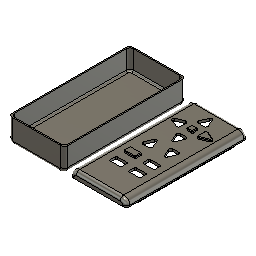
northreach_1_v2 (Autodesk Fusion 360 design; units mm, degrees)
Autodesk Fusion 360 part; units mm, degrees
note: some values were not read from the file. Set by a fixed rule: which sketch regions a step uses.
sketch "MainBodyBase" plane through (0, 0, 0) normal (0, 1, 0) x (1, 0, 0)
  line L0 (-22.5, 50) -> (22.5, 50)
  line L1 (22.5, 50) -> (22.5, -50)
  line L2 (22.5, -50) -> (-22.5, -50)
  line L3 (-22.5, -50) -> (-22.5, 50)
  line L4 (-22.5, 50) -> (22.5, -50) construction
  line L5 (22.5, 50) -> (-22.5, -50) construction
  line L6 (-23.5, 51) -> (23.5, 51)
  line L7 (23.5, 51) -> (23.5, -51)
  line L8 (23.5, -51) -> (-23.5, -51)
  line L9 (-23.5, -51) -> (-23.5, 51)
  line L10 (-23.5, 51) -> (23.5, -51) construction
  line L11 (23.5, 51) -> (-23.5, -51) construction
  dimension "d1" = 45
  dimension "d2" = 100
  dimension "d3" = 47
  dimension "d4" = 102
  constraint horizontal L0
  constraint perpendicular L0 L1
  constraint parallel L0 L2
  constraint parallel L1 L3
  constraint coincident L4 origin
  constraint coincident L5 origin
  constraint horizontal L6
  constraint perpendicular L6 L7
  constraint parallel L6 L8
  constraint parallel L7 L9
  constraint coincident L10 origin
  constraint coincident L11 origin
  measures "d1" distance of L1.end L2.end
  measures "d2" distance of L0.end L1.end
  measures "d3" distance of L7.end L8.end
  measures "d4" distance of L6.end L7.end
extrude "Extrude1" add sketch "MainBodyBase" along normal blind 3 contours L0 L1 L2 L3 makes body 1
extrude "Extrude2" add sketch "MainBodyBase" along normal blind 20 bodies 1
fillet "Fillet1" radius 4 2 edges at (-23.5, 0, 0) (23.5, 0, 0) on bodies 1
sketch "TopCoverBase" plane through (0, 0, 0) normal (0, 1, 0) x (1, 0, 0)
  line L0 (46.5, 51) -> (93.5, 51)
  line L1 (93.5, 51) -> (93.5, -51)
  line L2 (93.5, -51) -> (46.5, -51)
  line L3 (46.5, -51) -> (46.5, 51)
  line L4 (46.5, 51) -> (93.5, -51) construction
  line L5 (93.5, 51) -> (46.5, -51) construction
  line L6 (48.5, 50) -> (91.5, 50)
  line L7 (91.5, 50) -> (91.5, -50)
  line L8 (91.5, -50) -> (48.5, -50)
  line L9 (48.5, -50) -> (48.5, 50)
  line L10 (48.5, 50) -> (91.5, -50) construction
  line L11 (91.5, 50) -> (48.5, -50) construction
  line L12 (47.5, 50) -> (47.5, -50)
  line L13 (48.5, -50) -> (48.5, 50)
  line L14 (92.5, -50) -> (92.5, 50)
  line L15 (91.5, 50) -> (91.5, -50)
  line L16 (47.5, 39.9985) -> (48.5, 39.9985)
  line L17 (47.5, -40) -> (48.5, -40)
  line L18 (91.5, -40) -> (92.5, -40)
  line L19 (91.5, 39.9985) -> (92.5, 39.9985)
  point P0 (70, 0)
  point P1 (70, 0)
  dimension "d22" = 47
  dimension "d23" = 102
  dimension "d24" = 43
  dimension "d25" = 100
  constraint horizontal L0
  constraint perpendicular L0 L1
  constraint parallel L0 L2
  constraint parallel L1 L3
  constraint coincident L4 P1
  constraint coincident L5 P1
  constraint horizontal L6
  constraint perpendicular L6 L7
  constraint parallel L6 L8
  constraint parallel L7 L9
  constraint coincident L10 P1
  constraint coincident L11 P1
  constraint coincident P1 P0
  constraint vertical L12
  constraint vertical L13
  constraint vertical L14
  constraint vertical L15
  constraint coincident L12 L16.start
  constraint coincident L13 L16.end
  constraint perpendicular L13 L16
  constraint coincident L12 L17.start
  constraint coincident L13 L17.end
  constraint perpendicular L13 L17
  constraint coincident L15 L18.start
  constraint coincident L14 L18.end
  constraint perpendicular L14 L18
  constraint coincident L7 L19.start
  constraint coincident L14 L19.end
  constraint perpendicular L14 L19
  measures "d22" distance of L1.end L2.end
  measures "d23" distance of L0.end L1.end
  measures "d24" distance of L7.end L8.end
  measures "d25" distance of L6.end L7.end
extrude "Extrude7" add sketch "TopCoverBase" along normal blind 2 separate body contours L6 L7 L8 L9 L13 L15 makes body 2
extrude "Extrude8" add sketch "TopCoverBase" along normal blind 6 contours L0 L1 L2 L3 | L9 L12 L13 L16 L17 | L7 L14 L15 L18 L19 bodies 2
extrude "Extrude9" add sketch "TopCoverBase" along normal blind 7.5 contours L9 L12 L13 L16 L17 | L7 L14 L15 L18 L19 bodies 2
fillet "Fillet2" radius 5 2 edges at (46.5, 0, 0) (93.5, 0, 0) on bodies 2
fillet "Fillet2" radius 3 2 edges at (91.5, 2, 0) (48.5, 2, 0) on bodies 2
move_body "Move1" bodies 2 to x (-1, 0, 0) y (0, -1, 0) z (0, 0, 1) at (122, 7.5, 0)
sketch "ButtonHoles" plane through (0, 7.5, 0) normal (0, 1, 0) x (-1, 0, 0)
  line L0 (-33.5, -51) -> (-33.5, 51)
  line L1 (-33.5, 51) -> (-70.5, 51)
  line L2 (-70.5, 51) -> (-70.5, -51)
  line L3 (-70.5, -51) -> (-33.5, -51)
  arc A0 (-39, 16.25) -> (-39.75, 17) centre (-39.75, 16.25) ccw
  line L4 (-49, 14) -> (-55, 14)
  arc A1 (-50.25, -30.5) -> (-49.5, -29.75) centre (-50.25, -29.75) ccw
  line L5 (-39.75, 11) -> (-48.25, 11)
  arc A2 (-55, 16.25) -> (-55.75, 17) centre (-55.75, 16.25) ccw
  line L6 (-46, 14) -> (-42, 14)
  line L7 (-53.75, -30.5) -> (-50.25, -30.5)
  line L8 (-54.5, -26.25) -> (-54.5, -29.75)
  line L9 (-49.5, -25.5) -> (-54.5, -30.5) construction
  arc A3 (-65, 11.75) -> (-64.25, 11) centre (-64.25, 11.75) ccw
  line L10 (-65, 11) -> (-55, 17) construction
  line L11 (-39, 16.25) -> (-39, 11.75)
  line L12 (-48.25, 17) -> (-39.75, 17)
  line L13 (-65, 23) -> (-55, 29) construction
  line L14 (-62, 26) -> (-58, 26)
  line L15 (-41.4931, 3.0384) -> (-46.5069, 3.0384)
  line L16 (-39, 28.25) -> (-39, 23.75)
  line L17 (-55.75, 23) -> (-64.25, 23)
  arc A4 (-39.75, 11) -> (-39, 11.75) centre (-39.75, 11.75) ccw
  line L18 (-49, 23) -> (-39, 29) construction
  line L19 (-39.75, 23) -> (-48.25, 23)
  arc A5 (-64.25, 29) -> (-65, 28.25) centre (-64.25, 28.25) ccw
  line L20 (-55, 11) -> (-65, 17) construction
  arc A6 (-49.5, -26.25) -> (-50.25, -25.5) centre (-50.25, -26.25) ccw
  line L21 (-49, 11) -> (-39, 17) construction
  arc A7 (-49, 23.75) -> (-48.25, 23) centre (-48.25, 23.75) ccw
  line L22 (-47.8763, 0.9617) -> (-45.1295, -5.4475)
  line L23 (-55, 28.25) -> (-55, 23.75)
  line L24 (-49, 26) -> (-55, 26)
  arc A8 (-47.8763, 0.9617) -> (-46.5069, 3.0384) centre (-46.5069, 1.5486) cw
  line L25 (-42.8705, -5.4475) -> (-40.1237, 0.9617)
  line L26 (-55, 23) -> (-65, 29) construction
  arc A9 (-55, 28.25) -> (-55.75, 29) centre (-55.75, 28.25) ccw
  line L27 (-54.5, -25.5) -> (-49.5, -30.5) construction
  line L28 (-65, 23.75) -> (-65, 28.25)
  line L29 (-46, 26) -> (-42, 26)
  line L30 (-64.25, 17) -> (-55.75, 17)
  line L31 (-39, 11) -> (-49, 17) construction
  arc A10 (-54.5, -29.75) -> (-53.75, -30.5) centre (-53.75, -29.75) ccw
  line L32 (-50.25, -25.5) -> (-53.75, -25.5)
  arc A11 (-53.75, -25.5) -> (-54.5, -26.25) centre (-53.75, -26.25) ccw
  line L33 (-44, 12) -> (-44, 16)
  arc A12 (-49, 11.75) -> (-48.25, 11) centre (-48.25, 11.75) ccw
  line L34 (-60, 24) -> (-60, 28)
  line L35 (-65, 11.75) -> (-65, 16.25)
  line L36 (-44, 24) -> (-44, 28)
  line L37 (-39, 23) -> (-49, 29) construction
  line L38 (-62, 14) -> (-58, 14)
  line L39 (-49.5, -29.75) -> (-49.5, -26.25)
  line L40 (-60, 12) -> (-60, 16)
  arc A13 (-64.25, 17) -> (-65, 16.25) centre (-64.25, 16.25) ccw
  line L41 (-49, 11.75) -> (-49, 16.25)
  arc A14 (-65, 23.75) -> (-64.25, 23) centre (-64.25, 23.75) ccw
  arc A15 (-41.4931, 3.0384) -> (-40.1237, 0.9617) centre (-41.4931, 1.5486) cw
  arc A16 (-48.25, 17) -> (-49, 16.25) centre (-48.25, 16.25) ccw
  arc A17 (-39, 28.25) -> (-39.75, 29) centre (-39.75, 28.25) ccw
  line L42 (-44, -6.1923) -> (-44, 3.0384)
  line L43 (-49, 23.75) -> (-49, 28.25)
  arc A18 (-55.75, 11) -> (-55, 11.75) centre (-55.75, 11.75) ccw
  arc A19 (-39.75, 23) -> (-39, 23.75) centre (-39.75, 23.75) ccw
  line L44 (-48.25, 29) -> (-39.75, 29)
  line L45 (-55.75, 11) -> (-64.25, 11)
  arc A20 (-48.25, 29) -> (-49, 28.25) centre (-48.25, 28.25) ccw
  arc A21 (-42.8705, -5.4475) -> (-45.1295, -5.4475) centre (-44, -4.9635) cw
  line L46 (-64.25, 29) -> (-55.75, 29)
  arc A22 (-55.75, 23) -> (-55, 23.75) centre (-55.75, 23.75) ccw
  line L47 (-55, 16.25) -> (-55, 11.75)
  line L48 (-42, 16) -> (-46, 16) construction
  line L49 (-46, 16) -> (-46, 12) construction
  line L50 (-46, 12) -> (-42, 12) construction
  line L51 (-42, 12) -> (-42, 16) construction
  line L52 (-42, 28) -> (-46, 28) construction
  line L53 (-46, 28) -> (-46, 24) construction
  line L54 (-46, 24) -> (-42, 24) construction
  line L55 (-42, 24) -> (-42, 28) construction
  line L56 (-58, 16) -> (-62, 16) construction
  line L57 (-62, 16) -> (-62, 12) construction
  line L58 (-62, 12) -> (-58, 12) construction
  line L59 (-58, 12) -> (-58, 16) construction
  line L60 (-58, 28) -> (-62, 28) construction
  line L61 (-62, 28) -> (-62, 24) construction
  line L62 (-62, 24) -> (-58, 24) construction
  line L63 (-58, 24) -> (-58, 28) construction
  line L64 (-44, -1.577) -> (-60, -1.577)
  line L65 (-41.4931, 3.0384) -> (-46.5069, 3.0384)
  line L66 (-44, -6.1923) -> (-44, 3.0384)
  arc A23 (-47.8763, 0.9617) -> (-46.5069, 3.0384) centre (-46.5069, 1.5486) cw
  arc A24 (-42.8705, -5.4475) -> (-45.1295, -5.4475) centre (-44, -4.9635) cw
  line L67 (-42.8705, -5.4475) -> (-40.1237, 0.9617)
  arc A25 (-41.4931, 3.0384) -> (-40.1237, 0.9617) centre (-41.4931, 1.5486) cw
  line L68 (-47.8763, 0.9617) -> (-45.1295, -5.4475)
  line L69 (-62.5069, -6.1923) -> (-57.4931, -6.1923)
  line L70 (-60, 3.0384) -> (-60, -6.1923)
  arc A26 (-56.1237, -4.1156) -> (-57.4931, -6.1923) centre (-57.4931, -4.7025) cw
  arc A27 (-61.1295, 2.2936) -> (-58.8705, 2.2936) centre (-60, 1.8095) cw
  line L71 (-61.1295, 2.2936) -> (-63.8763, -4.1156)
  arc A28 (-62.5069, -6.1923) -> (-63.8763, -4.1156) centre (-62.5069, -4.7025) cw
  line L72 (-56.1237, -4.1156) -> (-58.8705, 2.2936)
  line L73 (-52, -11.2693) -> (-52, -20.5)
  line L74 (-53.1295, -12.0141) -> (-55.8763, -18.4233)
  arc A29 (-48.1237, -18.4233) -> (-49.4931, -20.5) centre (-49.4931, -19.0102) cw
  line L75 (-48.1237, -18.4233) -> (-50.8705, -12.0141)
  arc A30 (-54.5069, -20.5) -> (-55.8763, -18.4233) centre (-54.5069, -19.0102) cw
  line L76 (-54.5069, -20.5) -> (-49.4931, -20.5)
  arc A31 (-53.1295, -12.0141) -> (-50.8705, -12.0141) centre (-52, -12.4982) cw
  line L77 (-68.7307, -28) -> (-59.5, -28)
  line L78 (-67.9859, -29.1295) -> (-61.5767, -31.8763)
  arc A32 (-61.5767, -24.1237) -> (-59.5, -25.4931) centre (-60.9898, -25.4931) cw
  line L79 (-61.5767, -24.1237) -> (-67.9859, -26.8705)
  arc A33 (-59.5, -30.5069) -> (-61.5767, -31.8763) centre (-60.9898, -30.5069) cw
  line L80 (-59.5, -30.5069) -> (-59.5, -25.4931)
  arc A34 (-67.9859, -29.1295) -> (-67.9859, -26.8705) centre (-67.5019, -28) cw
  line L81 (-35.2693, -28) -> (-44.5, -28)
  line L82 (-36.0141, -26.8705) -> (-42.4233, -24.1237)
  arc A35 (-42.4233, -31.8763) -> (-44.5, -30.5069) centre (-43.0102, -30.5069) cw
  line L83 (-42.4233, -31.8763) -> (-36.0141, -29.1295)
  arc A36 (-44.5, -25.4931) -> (-42.4233, -24.1237) centre (-43.0102, -25.4931) cw
  line L84 (-44.5, -25.4931) -> (-44.5, -30.5069)
  arc A37 (-36.0141, -26.8705) -> (-36.0141, -29.1295) centre (-36.4981, -28) cw
  line L85 (-52, -44.7307) -> (-52, -35.5)
  line L86 (-50.8705, -43.9859) -> (-48.1237, -37.5767)
  arc A38 (-55.8763, -37.5767) -> (-54.5069, -35.5) centre (-54.5069, -36.9898) cw
  line L87 (-55.8763, -37.5767) -> (-53.1295, -43.9859)
  arc A39 (-49.4931, -35.5) -> (-48.1237, -37.5767) centre (-49.4931, -36.9898) cw
  line L88 (-49.4931, -35.5) -> (-54.5069, -35.5)
  arc A40 (-50.8705, -43.9859) -> (-53.1295, -43.9859) centre (-52, -43.5019) cw
  point P0 (-44, 26)
  point P1 (-60, 14)
  point P2 (-44, 3.0384)
  point P3 (-52.0007, 8.4459)
  point P4 (-44, 14)
  point P5 (-41.5, 10)
  point P6 (-44, 14)
  point P7 (-41.5, 22)
  point P8 (-44, 26)
  point P9 (-52, 14)
  point P10 (-44, -1.577)
  point P11 (-52, 26)
  point P12 (-60, 14)
  point P13 (-52, -28)
  point P14 (-60, 26)
  point P15 (-60, 26)
  point P16 (-52, -1.577)
  point P17 (-44, 3.0384)
  point P18 (-44, -1.577)
  point P19 (-44, -1.577)
  point P20 (-60, -6.1923)
  point P21 (-60, -1.577)
  point P22 (-60, -1.577)
  point P23 (-52, -15.8847)
  point P24 (-52, -20.5)
  point P25 (-52, -15.8847)
  point P26 (-52, -15.8847)
  point P27 (-64.1153, -28)
  point P28 (-59.5, -28)
  point P29 (-64.1153, -28)
  point P30 (-64.1153, -28)
  point P31 (-39.8847, -28)
  point P32 (-44.5, -28)
  point P33 (-39.8847, -28)
  point P34 (-39.8847, -28)
  point P35 (-52, -40.1153)
  point P36 (-52, -35.5)
  point P37 (-52, -40.1153)
  point P38 (-52, -40.1153)
  dimension "d46" = 3
  dimension "d47" = 0
  dimension "d50" = 3
  dimension "d51" = 0
  dimension "d48" = 3
  dimension "d49" = 0
  dimension "d52" = 3
  dimension "d53" = 0
  dimension "d55" = 0.75
  dimension "d56" = 10
  dimension "d57" = 6
  dimension "d58" = 10
  dimension "d59" = 6
  dimension "d60" = 6
  dimension "d61" = 0.75
  dimension "d62" = 10
  dimension "d63" = 6
  dimension "d64" = 10
  dimension "d65" = 6
  dimension "d66" = 6
  dimension "d67" = 0.75
  text T0 "1" font "Arial" height 3 align centre middle in box 4 x 4 at (-42, 16) x (-1, 0) y (0, -1) spacing 1
  text T1 "3" font "Arial" height 3 align centre middle in box 4 x 4 at (-42, 28) x (-1, 0) y (0, -1) spacing 1
  text T2 "2" font "Arial" height 3 align centre middle in box 4 x 4 at (-58, 16) x (-1, 0) y (0, -1) spacing 1
  text T3 "4" font "Arial" height 3 align centre middle in box 4 x 4 at (-58, 28) x (-1, 0) y (0, -1) spacing 1
  constraint horizontal L32
  constraint perpendicular L8 L32
  constraint parallel L7 L32
  constraint parallel L8 L39
  constraint coincident P13 L9
  constraint coincident P13 L27
  constraint coincident L9.end L7
  constraint coincident L9.end L8
  constraint tangent L7 A10
  constraint tangent L8 A10
  constraint coincident L27.end L7
  constraint coincident L27.end L39
  constraint tangent A1 L7
  constraint tangent A1 L39
  constraint equal A1 A10
  constraint coincident L9.start L39
  constraint coincident L9.start L32
  constraint tangent A6 L39
  constraint tangent A6 L32
  constraint equal A6 A10
  constraint coincident L27.start L32
  constraint coincident L27.start L8
  constraint tangent L32 A11
  constraint tangent L8 A11
  constraint equal A10 A11
  constraint tangent L15 A8
  constraint tangent L22 A8
  constraint tangent L15 A15
  constraint tangent L25 A15
  constraint tangent L22 A21
  constraint tangent L25 A21
  constraint midpoint P17 L15
  constraint midpoint L42.start A21
  constraint coincident P17 P2
  constraint perpendicular L15 L42
  constraint midpoint P19 L42
  constraint horizontal L45
  constraint perpendicular L35 L45
  constraint parallel L30 L45
  constraint parallel L35 L47
  constraint horizontal L5
  constraint perpendicular L5 L41
  constraint parallel L5 L12
  constraint parallel L11 L41
  constraint midpoint P9 L4
  constraint tangent L11 A4
  constraint tangent L5 A4
  constraint tangent A0 L11
  constraint tangent A0 L12
  constraint equal A0 A4
  constraint coincident L4.start L41
  constraint tangent L12 A16
  constraint tangent L41 A16
  constraint equal A4 A16
  constraint tangent L5 A12
  constraint tangent A12 L41
  constraint equal A4 A12
  constraint coincident L4.end L47
  constraint coincident L20.start L47
  constraint tangent A18 L45
  constraint tangent A18 L47
  constraint equal A4 A18
  constraint coincident L10.end L47
  constraint tangent A2 L47
  constraint tangent A2 L30
  constraint equal A2 A4
  constraint coincident L20.end L30
  constraint tangent L30 A13
  constraint tangent L35 A13
  constraint equal A4 A13
  constraint tangent A3 L45
  constraint tangent A3 L35
  constraint equal A3 A4
  constraint horizontal L17
  constraint perpendicular L17 L28
  constraint parallel L17 L46
  constraint parallel L23 L28
  constraint horizontal L19
  constraint perpendicular L19 L43
  constraint parallel L19 L44
  constraint parallel L16 L43
  constraint midpoint P11 L24
  constraint tangent L16 A19
  constraint tangent L19 A19
  constraint tangent L16 A17
  constraint tangent A17 L44
  constraint equal A17 A19
  constraint coincident L24.start L43
  constraint tangent L44 A20
  constraint tangent L43 A20
  constraint equal A19 A20
  constraint tangent L19 A7
  constraint tangent A7 L43
  constraint equal A7 A19
  constraint coincident L24.end L23
  constraint coincident L26.start L23
  constraint tangent L17 A22
  constraint tangent L23 A22
  constraint equal A19 A22
  constraint coincident L13.end L23
  constraint tangent L23 A9
  constraint tangent A9 L46
  constraint equal A9 A19
  constraint coincident L26.end L46
  constraint tangent A5 L46
  constraint tangent A5 L28
  constraint equal A5 A19
  constraint tangent L17 A14
  constraint tangent L28 A14
  constraint equal A14 A19
  constraint midpoint L33.start L50
  constraint midpoint L33.end L48
  constraint midpoint L6.start L49
  constraint midpoint L6.end L51
  constraint midpoint P6 L6
  constraint midpoint L40.start L58
  constraint midpoint L40.end L56
  constraint midpoint L38.start L57
  constraint midpoint L38.end L59
  constraint midpoint P1 L38
  constraint midpoint L36.start L54
  constraint midpoint L36.end L52
  constraint midpoint L29.start L53
  constraint midpoint L29.end L55
  constraint midpoint P8 L29
  constraint midpoint L34.start L62
  constraint midpoint L34.end L60
  constraint midpoint L14.start L61
  constraint midpoint L14.end L63
  constraint midpoint P15 L14
  constraint coincident P19 P18
  constraint tangent L65 A23
  constraint tangent A23 L68
  constraint tangent L65 A25
  constraint tangent L67 A25
  constraint tangent A24 L68
  constraint tangent A24 L67
  constraint midpoint P17 L65
  constraint midpoint L42.start A24
  constraint perpendicular L65 L66
  constraint midpoint P19 L66
  constraint tangent L69 A26
  constraint tangent A26 L72
  constraint tangent L69 A28
  constraint tangent L71 A28
  constraint tangent A27 L72
  constraint tangent A27 L71
  constraint midpoint P20 L69
  constraint midpoint L70.start A27
  constraint coincident P20 L70.end
  constraint perpendicular L69 L70
  constraint midpoint P22 L70
  constraint coincident P22 P21
  constraint tangent A29 L76
  constraint tangent A29 L75
  constraint tangent A30 L76
  constraint tangent L74 A30
  constraint tangent L75 A31
  constraint tangent L74 A31
  constraint midpoint P24 L76
  constraint midpoint L73.start A31
  constraint coincident P24 L73.end
  constraint perpendicular L73 L76
  constraint midpoint P26 L73
  constraint coincident P26 P25
  constraint tangent A32 L80
  constraint tangent A32 L79
  constraint tangent A33 L80
  constraint tangent L78 A33
  constraint tangent L79 A34
  constraint tangent L78 A34
  constraint midpoint P28 L80
  constraint midpoint L77.start A34
  constraint coincident P28 L77.end
  constraint perpendicular L77 L80
  constraint midpoint P30 L77
  constraint coincident P30 P29
  constraint tangent A35 L84
  constraint tangent A35 L83
  constraint tangent A36 L84
  constraint tangent L82 A36
  constraint tangent L83 A37
  constraint tangent L82 A37
  constraint midpoint P32 L84
  constraint midpoint L81.start A37
  constraint coincident P32 L81.end
  constraint perpendicular L81 L84
  constraint midpoint P34 L81
  constraint coincident P34 P33
  constraint tangent A38 L88
  constraint tangent A38 L87
  constraint tangent A39 L88
  constraint tangent L86 A39
  constraint tangent L87 A40
  constraint tangent L86 A40
  constraint midpoint P36 L88
  constraint midpoint L85.start A40
  constraint coincident P36 L85.end
  constraint perpendicular L85 L88
  constraint midpoint P38 L85
  constraint coincident P38 P37
  measures "d55" radius of A10
  measures "d56" distance of L20.end L10.end
  measures "d57" distance of L20.end L10.start
  measures "d58" distance of L21.end L31.end
  measures "d59" distance of L21.start L31.end
  measures "d60" distance of L41 L47
  measures "d61" radius of A4
  measures "d62" distance of L13.end L26.end
  measures "d63" distance of L13.start L26.end
  measures "d64" distance of L37.end L18.end
  measures "d65" distance of L37.end L18.start
  measures "d66" distance of L23 L43
  measures "d67" radius of A19
extrude "Extrude10" cut sketch "ButtonHoles" sketch "ButtonHoles" against normal blind 32 contours A0 L5 L11 L12 A4 A12 L41 A16 | A1 L7 L8 A6 A10 L32 A11 L39 | A2 A3 L30 L35 A13 A18 L45 L47 | L15 L25 A15 L42 A21 L65 L66 A24 L67 A25 | L15 L22 A8 L42 L64 L65 L66 A23 L68 | L22 L42 A21 L64 L66 A24 L68 | L16 L19 A7 A17 L43 A19 L44 A20 | L17 A5 L23 A9 L28 A14 L46 A22 | L64 L69 L70 A26 L72 | L64 L70 A27 L72 | L69 L70 A27 L71 A28 | L73 A29 L75 L76 A31 | L73 L74 A30 L76 A31 | L77 A32 L79 L80 A34 | L77 L78 A33 L80 A34 | L81 A35 L83 L84 A37 | L81 L82 A36 L84 A37 | L85 A38 L87 L88 A40 | L85 L86 A39 L88 A40 of sketch 2 text T0 T1 T2 T3 bodies 2
fillet "Fillet4" radius 3 14 edges at (23.5, 12, 51) (22.3284, 1.1716, 51) (0, 0, 51) (-22.3284, 1.1716, 51) (-23.5, 12, 51) (-22.5, 11.5, 50) (22.5, 11.5, 50) (-23.5, 12, -51) (-22.3284, 1.1716, -51) (0, 0, -51) (22.3284, 1.1716, -51) (23.5, 12, -51) (22.5, 11.5, -50) (-22.5, 11.5, -50) on bodies 1
fillet "Fillet5" radius 3 10 edges at (28.5, 2, 51) (29.9645, 6.0355, 51) (52, 7.5, 51) (74.0355, 6.0355, 51) (75.5, 2, 51) (75.5, 2, -51) (74.0355, 6.0355, -51) (52, 7.5, -51) (29.9645, 6.0355, -51) (28.5, 2, -51) on bodies 2
fillet "Fillet6" radius 1.5 8 edges at (0, 3, -50) (-21.6213, 3, -49.1213) (-22.5, 3, 0) (-21.6213, 3, 49.1213) (0, 3, 50) (21.6213, 3, 49.1213) (22.5, 3, 0) (21.6213, 3, -49.1213) on bodies 1
sketch "TriangleButton" plane through (0, 0, 0) normal (0, 1, 0) x (1, 0, 0)
  line L0 (-60, 2.8999) -> (-60, -6.0539)
  line L1 (-61.0956, 2.1775) -> (-63.76, -4.0395)
  arc A0 (-56.24, -4.0395) -> (-57.5683, -6.0539) centre (-57.5683, -4.6087) cw
  line L2 (-56.24, -4.0395) -> (-58.9044, 2.1775)
  arc A1 (-62.4317, -6.0539) -> (-63.76, -4.0395) centre (-62.4317, -4.6087) cw
  line L3 (-62.4317, -6.0539) -> (-57.5683, -6.0539)
  arc A2 (-61.0956, 2.1775) -> (-58.9044, 2.1775) centre (-60, 1.7079) cw
  point P0 (-60, -1.577)
  point P1 (-60, -6.0539)
  point P2 (-60, -1.577)
  point P3 (-60, -1.577)
  constraint tangent A0 L3
  constraint tangent A0 L2
  constraint tangent A1 L3
  constraint tangent L1 A1
  constraint tangent L2 A2
  constraint tangent L1 A2
  constraint midpoint P1 L3
  constraint midpoint L0.start A2
  constraint coincident P1 L0.end
  constraint perpendicular L0 L3
  constraint midpoint P3 L0
  constraint coincident P3 P2
extrude "Extrude12" add sketch "TriangleButton" along normal blind 6 separate body makes body 3
move_body "Move7" bodies 3 to x (0, 0, 1) y (0, 1, 0) z (-1, 0, 0) at (-67.0351, 0, 60.9584)
move_body "Move8" bodies 3 to x (1, 0, 0) y (0, 1, 0) z (0, 0, 1) at (132.7274, 1.5, -28.9584)
move_body "Move9" bodies 3 to x (1, 0, 0) y (0, 1, 0) z (0, 0, 1) at (-127, 0, 0)
ref_plane "WorkPlane1" through (-62.8847, 3.5, -28) normal (0, 1, 0) x (0, 0, 1)
sketch "TriangleButtonLip" plane through (0, 3.5, 0) normal (0, 1, 0) x (1, 0, 0)
  line L0 (-65.3472, 24.24) -> (-59.1302, 26.9044)
  arc A0 (-59.1302, 26.9044) -> (-59.1302, 29.0956) centre (-59.5997, 28) ccw
  line L1 (-59.1302, 29.0956) -> (-65.3472, 31.76)
  arc A1 (-65.3472, 31.76) -> (-67.3615, 30.4317) centre (-65.9164, 30.4317) ccw
  line L2 (-67.3615, 30.4317) -> (-67.3615, 25.5683)
  arc A2 (-67.3615, 25.5683) -> (-65.3472, 24.24) centre (-65.9164, 25.5683) ccw
  line L3 (-58.7363, 30.0147) -> (-64.9533, 32.6791)
  arc A3 (-64.9533, 32.6791) -> (-68.3615, 30.4317) centre (-65.9164, 30.4317) ccw
  line L4 (-68.3615, 30.4317) -> (-68.3615, 25.5683)
  arc A4 (-68.3615, 25.5683) -> (-64.9533, 23.3209) centre (-65.9164, 25.5683) ccw
  line L5 (-64.9533, 23.3209) -> (-58.7363, 25.9853)
  arc A5 (-58.7363, 25.9853) -> (-58.7363, 30.0147) centre (-59.5997, 28) ccw
  dimension "d85" = 1
extrude "Extrude13" add sketch "TriangleButtonLip" along normal mid plane 1 bodies 3
move_body "Move10" bodies 3 to x (1, 0, 0) y (0, 1, 0) z (0, 0, 1) at (127, 0, 0)
move_body "Move11" bodies 3 to x (1, 0, 0) y (0, 1, 0) z (0, 0, 1) at (0, 1.5, 0)
fillet "Fillet7" radius 0.5 6 edges at (64.7613, 9, -30.4278) (60.288, 9, -31.6382) (59.6385, 9, -28) (60.288, 9, -24.3618) (64.7613, 9, -25.5722) (68.5922, 9, -28) on bodies 3
sketch "SquareButton" plane through (0, 0, 0) normal (0, 1, 0) x (1, 0, 0)
  line L0 (-80.3025, -0.575) -> (-83.6975, -0.575)
  line L1 (-84.425, -0.575) -> (-79.575, -5.425) construction
  line L2 (-79.575, -4.6975) -> (-79.575, -1.3025)
  line L3 (-79.575, -0.575) -> (-84.425, -5.425) construction
  arc A0 (-84.425, -4.6975) -> (-83.6975, -5.425) centre (-83.6975, -4.6975) ccw
  arc A1 (-79.575, -1.3025) -> (-80.3025, -0.575) centre (-80.3025, -1.3025) ccw
  arc A2 (-80.3025, -5.425) -> (-79.575, -4.6975) centre (-80.3025, -4.6975) ccw
  line L4 (-84.425, -1.3025) -> (-84.425, -4.6975)
  arc A3 (-83.6975, -0.575) -> (-84.425, -1.3025) centre (-83.6975, -1.3025) ccw
  line L5 (-83.6975, -5.425) -> (-80.3025, -5.425)
  point P0 (-82, -3)
  constraint horizontal L0
  constraint perpendicular L0 L4
  constraint parallel L0 L5
  constraint parallel L2 L4
  constraint coincident P0 L3
  constraint coincident P0 L1
  constraint coincident L3.end L5
  constraint coincident L3.end L4
  constraint tangent A0 L5
  constraint tangent A0 L4
  constraint coincident L1.end L5
  constraint coincident L1.end L2
  constraint tangent A2 L5
  constraint tangent L2 A2
  constraint equal A0 A2
  constraint coincident L3.start L2
  constraint coincident L3.start L0
  constraint tangent L2 A1
  constraint tangent L0 A1
  constraint equal A0 A1
  constraint coincident L1.start L0
  constraint coincident L1.start L4
  constraint tangent L0 A3
  constraint tangent L4 A3
  constraint equal A0 A3
extrude "Extrude14" add sketch "SquareButton" along normal blind 6 separate body makes body 4
ref_plane "WorkPlane2" through (-82, 2, 3) normal (0, 1, 0) x (1, 0, 0)
fillet "Fillet8" radius 0.5 8 edges at (-84.425, 6, 3) (-84.2119, 6, 5.2119) (-82, 6, 5.425) (-79.7881, 6, 5.2119) (-79.575, 6, 3) (-79.7881, 6, 0.7881) (-82, 6, 0.575) (-84.2119, 6, 0.7881) on bodies 4
sketch "SquareButtonLip" plane through (0, 2, 0) normal (0, 1, 0) x (1, 0, 0)
  line L0 (-84.425, -1.3025) -> (-84.425, -4.6975)
  arc A0 (-84.425, -4.6975) -> (-83.6975, -5.425) centre (-83.6975, -4.6975) ccw
  line L1 (-83.6975, -5.425) -> (-80.3025, -5.425)
  arc A1 (-83.6975, -0.575) -> (-84.425, -1.3025) centre (-83.6975, -1.3025) ccw
  arc A2 (-80.3025, -5.425) -> (-79.575, -4.6975) centre (-80.3025, -4.6975) ccw
  line L2 (-79.575, -4.6975) -> (-79.575, -1.3025)
  line L3 (-80.3025, -0.575) -> (-83.6975, -0.575)
  arc A3 (-79.575, -1.3025) -> (-80.3025, -0.575) centre (-80.3025, -1.3025) ccw
  arc A4 (-85.425, -4.6975) -> (-83.6975, -6.425) centre (-83.6975, -4.6975) ccw
  line L4 (-83.6975, -6.425) -> (-80.3025, -6.425)
  arc A5 (-80.3025, -6.425) -> (-78.575, -4.6975) centre (-80.3025, -4.6975) ccw
  line L5 (-78.575, -4.6975) -> (-78.575, -1.3025)
  arc A6 (-78.575, -1.3025) -> (-80.3025, 0.425) centre (-80.3025, -1.3025) ccw
  line L6 (-80.3025, 0.425) -> (-83.6975, 0.425)
  arc A7 (-83.6975, 0.425) -> (-85.425, -1.3025) centre (-83.6975, -1.3025) ccw
  line L7 (-85.425, -1.3025) -> (-85.425, -4.6975)
  dimension "d101" = 1
extrude "Extrude16" add sketch "SquareButtonLip" along normal mid plane 1 bodies 4
move_body "Move12" bodies 4 to x (1, 0, 0) y (0, 1, 0) z (0, 0, 1) at (134, 1.5, -31)
move_body "Move13" bodies 4 to x (1, 0, 0) y (0, 1, 0) z (0, 0, 1) at (0, 1.5, 0)
sketch "Sketch13" plane through (0, 0, 0) normal (0, 1, 0) x (1, 0, 0)
  line L0 (-84.8775, 15.09) -> (-93.1225, 15.09)
  arc A0 (-93.85, 15.8175) -> (-93.1225, 15.09) centre (-93.1225, 15.8175) ccw
  line L1 (-93.85, 15.8175) -> (-93.85, 20.1825)
  line L2 (-84.15, 15.09) -> (-93.85, 20.91) construction
  line L3 (-93.85, 15.09) -> (-84.15, 20.91) construction
  arc A1 (-93.1225, 20.91) -> (-93.85, 20.1825) centre (-93.1225, 20.1825) ccw
  arc A2 (-84.15, 20.1825) -> (-84.8775, 20.91) centre (-84.8775, 20.1825) ccw
  line L4 (-93.1225, 20.91) -> (-84.8775, 20.91)
  arc A3 (-84.8775, 15.09) -> (-84.15, 15.8175) centre (-84.8775, 15.8175) ccw
  line L5 (-90.94, 18) -> (-87.06, 18)
  line L6 (-89, 16.06) -> (-89, 19.94)
  line L7 (-84.15, 20.1825) -> (-84.15, 15.8175)
  line L8 (-87, 20) -> (-91, 20) construction
  line L9 (-91, 20) -> (-91, 16) construction
  line L10 (-91, 16) -> (-87, 16) construction
  line L11 (-87, 16) -> (-87, 20) construction
  point P0 (-89, 18)
  point P1 (-84.15, 18)
  point P2 (-89, 18)
  dimension "d104" = 3
  dimension "d105" = 0
  text T0 "2" font "Arial" height 3 align centre middle in box 4 x 4 at (-87, 20) x (-1, 0) y (0, -1) spacing 1
  constraint horizontal L0
  constraint perpendicular L0 L1
  constraint parallel L0 L4
  constraint parallel L1 L7
  constraint coincident P1 L7
  constraint coincident L2.start L7
  constraint tangent L0 A3
  constraint tangent A3 L7
  constraint coincident L3.end L7
  constraint tangent A2 L7
  constraint tangent A2 L4
  constraint coincident L2.end L4
  constraint tangent A1 L4
  constraint tangent L1 A1
  constraint tangent L0 A0
  constraint tangent A0 L1
  constraint midpoint P2 L5
extrude "Extrude17" add sketch "Sketch13" sketch "Sketch13" along normal blind 6 separate body of sketch 2 text T0 makes body 5
ref_plane "WorkPlane3" through (-89, 2, -18) normal (0, 1, 0) x (1, 0, 0)
sketch "Sketch14" plane through (0, 2, 0) normal (0, 1, 0) x (1, 0, 0)
  line L0 (-93.85, 20.1825) -> (-93.85, 15.8175)
  arc A0 (-93.85, 15.8175) -> (-93.1225, 15.09) centre (-93.1225, 15.8175) ccw
  line L1 (-93.1225, 15.09) -> (-84.8775, 15.09)
  arc A1 (-84.8775, 15.09) -> (-84.15, 15.8175) centre (-84.8775, 15.8175) ccw
  line L2 (-84.15, 15.8175) -> (-84.15, 20.1825)
  arc A2 (-84.15, 20.1825) -> (-84.8775, 20.91) centre (-84.8775, 20.1825) ccw
  line L3 (-84.8775, 20.91) -> (-93.1225, 20.91)
  arc A3 (-93.1225, 20.91) -> (-93.85, 20.1825) centre (-93.1225, 20.1825) ccw
  line L4 (-84.8775, 21.91) -> (-93.1225, 21.91)
  arc A4 (-93.1225, 21.91) -> (-94.85, 20.1825) centre (-93.1225, 20.1825) ccw
  line L5 (-94.85, 20.1825) -> (-94.85, 15.8175)
  arc A5 (-94.85, 15.8175) -> (-93.1225, 14.09) centre (-93.1225, 15.8175) ccw
  line L6 (-93.1225, 14.09) -> (-84.8775, 14.09)
  arc A6 (-84.8775, 14.09) -> (-83.15, 15.8175) centre (-84.8775, 15.8175) ccw
  line L7 (-83.15, 15.8175) -> (-83.15, 20.1825)
  arc A7 (-83.15, 20.1825) -> (-84.8775, 21.91) centre (-84.8775, 20.1825) ccw
  dimension "d111" = 1
extrude "Extrude18" add sketch "Sketch14" along normal mid plane 1 bodies 5
fillet "Fillet9" radius 0.5 8 edges at (-89, 6, -20.91) (-93.6369, 6, -20.6969) (-93.85, 6, -18) (-93.6369, 6, -15.3031) (-89, 6, -15.09) (-84.3631, 6, -15.3031) (-84.15, 6, -18) (-84.3631, 6, -20.6969) on bodies 5
move_body "Move14" bodies 5 to x (1, 0, 0) y (0, 1, 0) z (0, 0, 1) at (133, 1.5, 32)
move_body "Move15" bodies 5 to x (1, 0, 0) y (0, 1, 0) z (0, 0, 1) at (0, 1.5, 0)
equation "d47 = '1'"
equation "d51 = '3'"
equation "d49 = '2'"
equation "d53 = '4'"
equation "d105 = '2'"
named bodies: "MainBody", "TopCover", "TriangleButton", "SquareButton", "RectangleButton"
